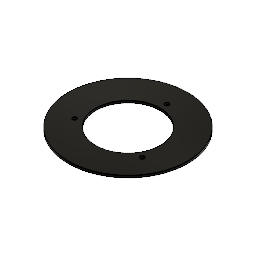
Isolator Plate v1 (Autodesk Fusion 360 design; units mm, degrees)
Autodesk Fusion 360 part; units mm, degrees
sketch "Sketch1" plane through (0, 0, 0) normal (0, 1, 0) x (1, 0, 0)
  circle A0 centre (0, 0) radius 14
  circle A1 centre (0, 0) radius 17 construction
  circle A2 centre (0, 0) radius 26
  arc A3 (14.7224, -8.5) -> (17, 0) centre (0, 0) ccw
  line L0 (0, 0) -> (14.7224, -8.5) construction
  line L1 (0, 0) -> (17, 0) construction
  circle A4 centre (14.7224, -8.5) radius 0.9
  circle A5 centre (0, 17) radius 0.9
  circle A6 centre (-14.7224, -8.5) radius 0.9
  dimension "d1" = 28
  dimension "d2" = 34
  dimension "d3" = 52
  dimension "d4" = 30
  dimension "d5" = 1.8
  dimension "d7" = 360
  measures "d1" diameter of A0
  measures "d2" diameter of A1
  measures "d3" diameter of A2
  measures "d4" angle of L0 L1
  measures "d5" diameter of A4
extrude "Extrude1" add sketch "Sketch1" along normal blind 1
